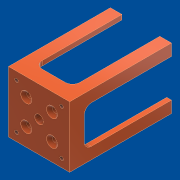
# Autodesk Inventor part: 901-4250 house
Saved by Autodesk Inventor 2018 (Build 220112000, 112)
## iProperties
Created: 2019-12-10
Part Number: 901-4250 house
Material: Generic
Document SubType Name: Modeling
Designer: Bunny320
Density: 1 g/cm^3
Appearance: Smooth - Light Orange
Author: Bunny320
## iProperties of the stored document 901-4250 house_3DPrint.ipt
Created: 2020-01-01
Part Number: 901-4250 house_3DPrint
Material: Generic
Document SubType Name: Modeling
Designer: Bunny320
Density: 1 g/cm^3
Appearance: Default
Author: Bunny320
Autodesk Inventor part; units mm, degrees
ref_plane "YZ Plane" through (0, 0, 0) normal (1, 0, 0) x (0, 1, 0)
ref_plane "XZ Plane" through (0, 0, 0) normal (0, 1, 0) x (-1, 0, 0)
ref_plane "XY Plane" through (0, 0, 0) normal (0, 0, 1) x (1, 0, 0)
sketch "Sketch1" plane through (0, 0, 0) normal (0, 1, 0) x (-1, 0, 0)
  line L0 (-21, 21) -> (21, 21)
  line L1 (21, 21) -> (21, -21)
  line L2 (21, -21) -> (-21, -21)
  line L3 (-21, -21) -> (-21, 21)
  line L4 (-21, 21) -> (21, -21) construction
  line L5 (21, 21) -> (-21, -21) construction
  point P0 (0, 0)
  dimension "d0" = 42
  constraints: 12 end point, 2 midpoint, 2 parallel, 2 perpendicular, 1 horizontal
  measures "d0" distance of L0.start L0.end
extrude "Extrusion1" add sketch "Sketch1" along normal blind 10
sketch "Sketch2" plane through (0, 10, 0) normal (0, 1, 0) x (1, 0, 0)
  line L0 (21, 21) -> (-21, 21) projected
  line L1 (-21, 21) -> (-13, 21)
  line L2 (-13, 21) -> (-13, 17.7482)
  line L3 (-17.7482, 13) -> (-21, 13)
  line L4 (-21, 13) -> (-21, 21)
  circle A0 centre (0, 0) radius 22
  dimension "d3" = 44
  dimension "d5" = 8
  constraints: 8 end point, 2 parallel, 2 perpendicular, 2 point on circle, 1 centre point, 1 coincident, 1 horizontal
  measures "d3" diameter of A0
  measures "d5" distance between parallel lines of L4 L2
extrude "Extrusion2" add sketch "Sketch2" along normal blind 60 contours L2 A0 L3 L4 L0
sketch "Sketch3" plane through (0, 0, 0) normal (0, 1, 0) x (-1, 0, 0)
  line L0 (-8.8388, 8.8388) -> (8.8388, 8.8388)
  line L1 (8.8388, 8.8388) -> (8.8388, -8.8388)
  line L2 (8.8388, -8.8388) -> (-8.8388, -8.8388)
  line L3 (-8.8388, -8.8388) -> (-8.8388, 8.8388)
  line L4 (-8.8388, 8.8388) -> (8.8388, -8.8388) construction
  line L5 (8.8388, 8.8388) -> (-8.8388, -8.8388) construction
  point P0 (0, 0)
  dimension "d11" = 25
  constraints: 12 end point, 2 midpoint, 2 parallel, 2 perpendicular, 1 coincident, 1 horizontal
  measures "d11" distance of L0.start L1.end
hole "Hole1" at (-8.8388, 0, -8.8388) direction (0, 1, 0) diameter 3.4 end through all countersink diameter 7.5 countersink angle 90 clearance for "Countersunk Flat Head Hex Socket Screw DIN EN ISO 10642" size "M3" standard "DIN"
fillet "Fillet1" radius 5 2 edges at (-13, 10, -19.3741) (-19.3741, 10, -13)
fillet "Fillet1" radius 2 1 edges at (-15.5563, 10, -15.5563)
sketch "Sketch5" plane through (0, 70, 0) normal (0, 1, 0) x (1, 0, 0)
  point P0 (0, 0)
  point P1 (-17.5, 17.5)
  dimension "d27" = 17.5
  dimension "d28" = 17.5
  measures "d27" horizontal distance of point (0, 0) point (-17.5, 17.5)
  measures "d28" horizontal distance of point (0, 0) point (-17.5, 17.5)
hole "Hole3" at (-17.5, 70, -17.5) direction (0, -1, 0) diameter 2.459 depth 20 tip angle 118 thread size "M3x0.5" class "6H" standard "ISO Metric profile"
sketch "Sketch4" plane through (0, 0, 0) normal (0, 1, 0) x (-1, 0, 0)
  line L0 (-15.5, 15.5) -> (15.5, 15.5)
  line L1 (15.5, 15.5) -> (15.5, -15.5)
  line L2 (15.5, -15.5) -> (-15.5, -15.5)
  line L3 (-15.5, -15.5) -> (-15.5, 15.5)
  line L4 (-15.5, 15.5) -> (15.5, -15.5) construction
  line L5 (15.5, 15.5) -> (-15.5, -15.5) construction
  point P0 (0, 0)
  dimension "d19" = 31
  constraints: 12 end point, 2 midpoint, 2 parallel, 2 perpendicular, 1 coincident, 1 horizontal
  measures "d19" distance of L0.start L0.end
hole "Hole2" at (-15.5, 0, -15.5) direction (0, 1, 0) diameter 2.459 depth 15 tip angle 118 thread size "M3x0.5" class "6H" standard "ISO Metric profile"
pattern_circular "Circular Pattern1" count 4 over 360 about axis through (0, -10, 0) along (0, 1, 0) of "Extrusion2", "Hole1", "Hole2", "Hole3", "Fillet1"
sketch "Sketch6" plane through (0, 10, 0) normal (0, 1, 0) x (1, 0, 0)
  point P0 (0, 0)
  point P1 (0, 0)
  constraints: 1 coincident
hole "Hole4" at (0, 10, 0) direction (0, -1, 0) diameter 6 end through all counterbore diameter 12 counterbore depth 2
equation "\"d28\" = d27"
body "Solid1"
